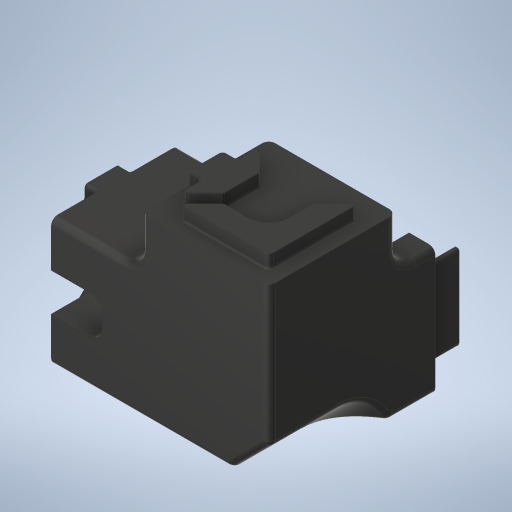
# Autodesk Inventor part: Exterior Frame Corner
Saved by Autodesk Inventor 2024 (Build 280153000, 153)
## iProperties
Category: PARTsolutions
Company: MISUMI
Created: 2024-08-20
Part Number: Exterior Frame Corner
Material: ABS Plastic
Catalog Web Link: www.cadenas.de
Description: NFS5-2020, NFSB5-2020, HFS5-2020, HFSB5-2020, CAF5-2020, HFSY5-2020, NFSF5-2020, HFSF5-2020, HFSFB5-2020, NFST5-2020, HFST5-2020, HFSTB5-2020, HFSH5-2020, HFSC5-2020-HFS5 Series Aluminum Extrusions 20 Square -1 Slot-
Vendor: MISUMI
Document SubType Name: Modeling
Designer: psAdmin
Manufacturer: MISUMI
Mass: 240.688 g
Surface Area: 837.523 cm^2
Volume: 89.1436 cm^3
Density: 1.06 g/cm^3
Appearance: Smooth - Black
PSOL_IDENT_0: {$CADENAS_DATA/23d-libs/misumi/metric/38_al_extrusions_blackets/5/hfs5_2020.prj},681 {VTYP=3D},{NB=H
PSOL_IDENT_1: FSTB5-2020-456},{LINA=HFSTB5-2020-456},{NN=NFS5-2020, NFSB5-2020, HFS5-2020, HFSB5-2020, CAF5-2020,
PSOL_IDENT_2: HFSY5-2020, NFSF5-2020, HFSF5-2020, HFSFB5-2020, NFST5-2020, HFST5-2020, HFSTB5-2020, HFSH5-2020, HF
PSOL_IDENT_3: SC5-2020},{DATE=08.05.2023 08:39:06},{GEOMDATE=27.07.2021 03:20:00},{VERSION=},{LINEID=110},{WBVAR=L
PSOL_IDENT_4: ,ALT1,ALT2,ALT4,ALT5,CP5,DL5,DR5,ALT6,ALT9,ALT10,ALT11,HP6,NHL6,DL6,NHR6,DR6,ALT7,ALT8,NH9,AH,BH,CH,
PSOL_IDENT_5: DH,EH,NH10,AV,BV,CV,DV,EV,NH11,AP,BP,CP,DP,EP,ALT12,ALT13,Z,NH12,XA,XB,XC,XD,XE,NH13,YA,YB,YC,YD,YE,
PSOL_IDENT_6: ALT16,HP16,DL16,DR16,ALT17,HQ17,JLP,ALT20},{WBNUMERIC=L,NH9,AH,BH,CH,DH,EH,NH10,AV,BV,CV,DV,EV,NH11,
PSOL_IDENT_7: AP,BP,CP,DP,EP,NH12,XA,XB,XC,XD,XE,NH13,YA,YB,YC,YD,YE,HQ17,JLP}  {NB=HFSTB5-2020-456},{LINA=HFSTB5-
PSOL_IDENT_8: 2020-456},{KT=DUMMY},{PN=HFSTB5-2020-456},{TPS=HFSTB5-2020},{MAT=A6N01SS-T5 Aluminum Alloy or 6005A-
PSOL_IDENT_9: T5 Aluminum Alloy},{ST=Black Anodize},{FRMW=20},{FRMH=20},{FRD=4.2},{L=456},{MASS=0.53},{SA=196},{LX=
PSOL_IDENT_10: 0.808x10^4},{LY=0.808x10^4},{ALT1=},{M1=0},{DPL1=0},{DPR1=0},{ALT1PN=},{ALT2=},{ALT2ALG= '','w/o End
PSOL_IDENT_11: Tapping (Heli-Coil Insert)','LHP','with LHP (Tapping on the Left (Heli-Coil Insert))','RHP','with R
PSOL_IDENT_12: HP (Tapping on the Right (Heli-Coil Insert))','HPW','with HPW (Tapping on Both Ends (Heli-Coil Inser
PSOL_IDENT_13: t))' },{M2=0},{DP2=0},{ALT2PN=},{ALT4=},{ALT4ALG= '', 'w/o SC (High Precision Cut)', 'SC', 'with SC
PSOL_IDENT_14: (High Precision Cut)' },{ALT4PN=},{ALT5=},{ALT5ALG= '','w/o 45 Degree Cut','1','with 45 Degree Cut'
PSOL_IDENT_15: },{CP5=},{CP5ALG= '','N/A' },{DL5=},{DL5ALG= '','N/A' },{DR5=},{DR5ALG= '','N/A' },{FRMLALT5=0},{FRM
PSOL_IDENT_16: RALT5=0},{ALT5PN=},{ALT6=},{ALT6ALG= '','w/o Fastening Location Wrench Access Hole Alterations','1','
PSOL_IDENT_17: with Fastening Location Wrench Access Hole Alterations' },{ALT9=},{ALT9ALG= '','w/o Location Specifi
PSOL_IDENT_18: ed Wrench Access Hole Alteratons (Horizontal)','1','with Location Specified Wrench Access Hole Alter
PSOL_IDENT_19: atons (Horizontal)' },{ALT10=},{ALT10ALG= '','w/o Location Specified Wrench Access Hole Alteratons (
PSOL_IDENT_20: Vertical)','1','with Location Specified Wrench Access Hole Alteratons (Vertical)' },{ALT11=},{ALT11A
PSOL_IDENT_21: LG= '','w/o Location Specified Wrench Access Hole Alteratons (Crisscross)','1','with Location Specif
PSOL_IDENT_22: ied Wrench Access Hole Alteratons (Crisscross)' },{HP6=},{HP6ALG= '','N/A' },{NHL6=},{NHL6ALG= '','N
PSOL_IDENT_23: /A' },{DL6=},{DL6ALG= '','N/A' },{NHR6=},{NHR6ALG= '','N/A' },{DR6=},{DR6ALG= '','N/A' },{HL6=0.000}
PSOL_IDENT_24: ,{HL6D=0},{HR6=0.000},{HR6D=0},{J6=0},{J6D=0},{K6=0},{K6D=0},{DD6=0.00},{DD6ALG=0},{ALT7=},{ALT7ALG=
PSOL_IDENT_25: '','N/A' },{ALT8=},{ALT8ALG= '','N/A' },{ALT678PN=},{NH9=0},{NH9MAX=5},{NH9ALG=[0]},{AH=0.0},{AHMIN=
PSOL_IDENT_26: 7},{AHMAX=451},{AHALG=[0]},{BH=0.0},{BHMIN=2},{BHMAX=453},{BHALG=[0]},{CH=0.0},{CHMIN=2},{CHMAX=455}
PSOL_IDENT_27: ,{CHALG=[0]},{DH=0.0},{DHMIN=2},{DHMAX=457},{DHALG=[0]},{EH=0.0},{EHMIN=2},{EHMAX=449},{EHALG=[0]},{
PSOL_IDENT_28: NH10=0},{NH10MAX=5},{NH10ALG=[0]},{AV=0.0},{AVMIN=7},{AVMAX=451},{AVALG=[0]},{BV=0.0},{BVMIN=2},{BVM
PSOL_IDENT_29: AX=453},{BVALG=[0]},{CV=0.0},{CVMIN=2},{CVMAX=455},{CVALG=[0]},{DV=0.0},{DVMIN=2},{DVMAX=457},{DVALG=
PSOL_IDENT_30: [0]},{EV=0.0},{EVMIN=2},{EVMAX=449},{EVALG=[0]},{NH11=0},{NH11MAX=5},{NH11ALG=[0]},{AP=0.0},{APMIN=7
PSOL_IDENT_31: },{APMAX=451},{APALG=[0]},{BP=0.0},{BPMIN=2},{BPMAX=453},{BPALG=[0]},{CP=0.0},{CPMIN=2},{CPMAX=455},
PSOL_IDENT_32: {CPALG=[0]},{DP=0.0},{DPMIN=2},{DPMAX=457},{DPALG=[0]},{EP=0.0},{EPMIN=2},{EPMAX=449},{EPALG=[0]},{A
PSOL_IDENT_33: LT9PN=},{ALT10PN=},{ALT11PN=},{ALT91011PN=},{ALT12=},{ALT12ALG= '','w/o Counterbore Hole in Specifie
PSOL_IDENT_34: d Position (Vertical)','1','with Counterbore Hole in Specified Position (Vertical)' },{ALT13=},{ALT1
PSOL_IDENT_35: 3ALG= '','N/A' },{Z=},{ZALG= '','N/A' },{DD12=0.0},{DD112=0.0},{NH12=0},{NH12MAX=5},{NH12ALG=[0]},{X
PSOL_IDENT_36: A=0.0},{XAMIN=7},{XAMAX=451},{XAALG=[0]},{XB=0.0},{XBMIN=2},{XBMAX=453},{XBALG=[0]},{XC=0.0},{XCMIN=
PSOL_IDENT_37: 2},{XCMAX=455},{XCALG=[0]},{XD=0.0},{XDMIN=2},{XDMAX=457},{XDALG=[0]},{XE=0.0},{XEMIN=2},{XEMAX=449}
PSOL_IDENT_38: ,{XEALG=[0]},{NH13=0},{NH13MAX=5},{NH13ALG=[0]},{YA=0.0},{YAMIN=7},{YAMAX=451},{YAALG=[0]},{YB=0.0},
PSOL_IDENT_39: {YBMIN=2},{YBMAX=453},{YBALG=[0]},{YC=0.0},{YCMIN=2},{YCMAX=455},{YCALG=[0]},{YD=0.0},{YDMIN=2},{YDM
PSOL_IDENT_40: AX=457},{YDALG=[0]},{YE=0.0},{YEMIN=2},{YEMAX=449},{YEALG=[0]},{ALT12PN=},{ALT13PN=},{ALT1213PN=},{A
PSOL_IDENT_41: LT16=},{ALT16ALG= '','w/o M Type Hole Alteration','1','with M Type Hole Alteration' },{HP16=},{HP16A
PSOL_IDENT_42: LG= '','N/A' },{DL16=},{DL16ALG= '','N/A' },{DR16=},{DR16ALG= '','N/A' },{H116=0},{D16=0.0},{ALT16PN=
PSOL_IDENT_43: },{ALT17=},{ALT17ALG= '','w/o L Type Hole Alteration (Top)','1','with L Type Hole Alteration (Top)'
PSOL_IDENT_44: },{HQ17=0},{HQ17ALG=0},{JLP=0},{JLPMIN=4.9},{JLPMAX=0},{JLPALG=[0]},{L17=0},{D17=0.0},{ALT17PN=},{AL
PSOL_IDENT_45: T20=},{ALT20PN=},{ERRORALT01=OK},{ERRORALT02=OK},{ERRORALT05=OK},{ERRORALT06091=OK},{ERRORALT06092=O
PSOL_IDENT_46: K},{ERRORALT06093=OK},{ERRORALT06094=OK},{ERRORALT06101=OK},{ERRORALT06102=OK},{ERRORALT06103=OK},{E
PSOL_IDENT_47: RRORALT06104=OK},{ERRORALT06111=OK},{ERRORALT06112=OK},{ERRORALT06113=OK},{ERRORALT06114=OK},{ERRORA
PSOL_IDENT_48: LT06121=OK},{ERRORALT06122=OK},{ERRORALT06123=OK},{ERRORALT06124=OK},{ERRORALT06131=OK},{ERRORALT061
PSOL_IDENT_49: 32=OK},{ERRORALT06133=OK},{ERRORALT06134=OK},{ERRORALT0616=OK},{ERRORALT06171=OK},{ERRORALT06172=OK}
PSOL_IDENT_50: ,{ERRORALT06173=OK},{ERRORALT0911=OK},{ERRORALT0913=OK},{ERRORALT0916=OK},{ERRORALT0917=OK},{ERRORAL
PSOL_IDENT_51: T1011=OK},{ERRORALT1012=OK},{ERRORALT1016=OK},{ERRORALT1017=OK},{ERRORALT1112=OK},{ERRORALT1113=OK},
PSOL_IDENT_52: {ERRORALT1116=OK},{ERRORALT1117=OK},{ERRORALT1216=OK},{ERRORALT1217=OK},{ERRORALT1316=OK},{ERRORALT1
PSOL_IDENT_53: 317=OK},{ERRORALT1617=OK},{ERRORPN=},{TFW=5}
NB: HFSTB5-2020-456
NN: NFS5-2020, NFSB5-2020, HFS5-2020, HFSB5-2020, CAF5-2020, HFSY5-2020, NFSF5-2020, HFSF5-2020, HFSFB5-2020, NFST5-2020, HFST5-2020, HFSTB5-2020, HFSH5-2020, HFSC5-2020
NT: HFS5 Series Aluminum Extrusions 20 Square -1 Slot-
NBSYN: $PN.
LINA: HFSTB5-2020-456
CATALOG: Misumi
PN: HFSTB5-2020-456
TPS: HFSTB5-2020
MAT: A6N01SS-T5 Aluminum Alloy or 6005A-T5 Aluminum Alloy
ST: Black Anodize
L: 456
MASS: 0.53
SA: 196
LX: 0.808x10^4
LY: 0.808x10^4
ALT1: w/o End Tapping
M1: 0
DPL1: 0
DPR1: 0
ALT2: w/o End Tapping (Heli-Coil Insert)
M2: 0
DP2: 0
ALT4: w/o SC (High Precision Cut)
ALT5: w/o 45 Degree Cut
CP5: N/A
DL5: N/A
DR5: N/A
ALT6: w/o Fastening Location Wrench Access Hole Alterations
ALT9: w/o Location Specified Wrench Access Hole Alteratons (Horizontal)
ALT10: w/o Location Specified Wrench Access Hole Alteratons (Vertical)
ALT11: w/o Location Specified Wrench Access Hole Alteratons (Crisscross)
HP6: N/A
NHL6: N/A
DL6: N/A
NHR6: N/A
DR6: N/A
HL6D: 0
HR6D: 0
J6D: 0
K6D: 0
DD6: 0
ALT7: N/A
ALT8: N/A
NH9: 0
AH: 0
BH: 0
CH: 0
DH: 0
EH: 0
NH10: 0
AV: 0
BV: 0
CV: 0
DV: 0
EV: 0
NH11: 0
AP: 0
BP: 0
CP: 0
DP: 0
EP: 0
ALT12: w/o Counterbore Hole in Specified Position (Vertical)
ALT13: N/A
Z: N/A
DD12: 0
DD112: 0
NH12: 0
XA: 0
XB: 0
XC: 0
XD: 0
XE: 0
NH13: 0
YA: 0
YB: 0
YC: 0
YD: 0
YE: 0
ALT16: w/o M Type Hole Alteration
HP16: N/A
DL16: N/A
DR16: N/A
H116: 0
D16: 0
ALT17: w/o L Type Hole Alteration (Top)
HQ17: 0
JLP: 0
D17: 0
ALT20: w/o CW (End Face C Chamfering)
SUPPLIER: MISUMI
ARTICLENO: HFSTB5-2020-456
BOMINFO: HFSTB5-2020-456
CREATOR: CADENAS GmbH
Title: HFSTB5-2020-456
Author: Cadenas PARTsolutions
Comments: HFS5 Series Aluminum Extrusions 20 Square -1 Slot-
Autodesk Inventor part; units mm, degrees
ref_plane "YZ Plane" through (0, 0, 0) normal (1, 0, 0) x (0, 1, 0)
ref_plane "XZ Plane" through (0, 0, 0) normal (0, 1, 0) x (-1, 0, 0)
ref_plane "XY Plane" through (0, 0, 0) normal (0, 0, 1) x (1, 0, 0)
sketch "Sketch_64" plane through (0, 0, 0) normal (0, 0, 1) x (1, 0, 0)
  line L0 (-10, -3) -> (-10, -9)
  arc A0 (-10, -9) -> (-9, -10) centre (-9, -9) ccw
  line L1 (-9, -10) -> (9, -10)
  arc A1 (9, -10) -> (10, -9) centre (9, -9) ccw
  line L2 (10, -9) -> (10, 9)
  arc A2 (10, 9) -> (9, 10) centre (9, 9) ccw
  line L3 (9, 10) -> (3, 10)
  line L4 (3, 10) -> (3, 8)
  line L5 (3, 8) -> (6, 8)
  line L6 (6, 8) -> (6, 7.0607)
  line L7 (6, 7.0607) -> (2.9393, 4)
  line L8 (2.9393, 4) -> (0.5196, 4)
  line L9 (0.5196, 4) -> (0, 3.7)
  line L10 (0, 3.7) -> (-0.5196, 4)
  line L11 (-0.5196, 4) -> (-2.9393, 4)
  line L12 (-2.9393, 4) -> (-6, 7.0607)
  line L13 (-6, 7.0607) -> (-6, 8)
  line L14 (-6, 8) -> (-3, 8)
  line L15 (-3, 8) -> (-3, 10)
  line L16 (-3, 10) -> (-9, 10)
  arc A3 (-9, 10) -> (-10, 9) centre (-9, 9) ccw
  line L17 (-10, 9) -> (-10, 3)
  line L18 (-10, 3) -> (-8, 3)
  line L19 (-8, 3) -> (-8, 6)
  line L20 (-8, 6) -> (-7.0607, 6)
  line L21 (-7.0607, 6) -> (-4, 2.9393)
  line L22 (-4, 2.9393) -> (-4, 0.5196)
  line L23 (-4, 0.5196) -> (-3.7, 0)
  line L24 (-3.7, 0) -> (-4, -0.5196)
  line L25 (-4, -0.5196) -> (-4, -2.9393)
  line L26 (-4, -2.9393) -> (-7.0607, -6)
  line L27 (-7.0607, -6) -> (-8, -6)
  line L28 (-8, -6) -> (-8, -3)
  line L29 (-8, -3) -> (-10, -3)
  line L30 (-6, -7.2678) -> (-6, -7.5)
  arc A4 (-6, -7.5) -> (-5.5, -8) centre (-5.5, -7.5) ccw
  line L31 (-5.5, -8) -> (7, -8)
  arc A5 (7, -8) -> (8, -7) centre (7, -7) ccw
  line L32 (8, -7) -> (8, 5.5)
  arc A6 (8, 5.5) -> (7.5, 6) centre (7.5, 5.5) ccw
  line L33 (7.5, 6) -> (7.2678, 6)
  arc A7 (7.2678, 6) -> (6.9142, 5.8536) centre (7.2678, 5.5) ccw
  line L34 (6.9142, 5.8536) -> (4.1464, 3.0858)
  arc A8 (4.1464, 3.0858) -> (4, 2.7322) centre (4.5, 2.7322) ccw
  line L35 (4, 2.7322) -> (4, -1)
  arc A9 (1, -4) -> (4, -1) centre (1, -1) ccw
  line L36 (1, -4) -> (-2.7322, -4)
  arc A10 (-2.7322, -4) -> (-3.0858, -4.1464) centre (-2.7322, -4.5) ccw
  line L37 (-3.0858, -4.1464) -> (-5.8536, -6.9142)
  arc A11 (-5.8536, -6.9142) -> (-6, -7.2678) centre (-5.5, -7.2678) ccw
  circle A12 centre (0, 0) radius 5.65
  line L38 (5.65, -5.65) -> (-10, -5.65)
  line L39 (-10, -5.65) -> (-10, 10)
  line L40 (-10, 10) -> (5.65, 10)
  line L41 (5.65, 10) -> (5.65, -5.65)
  point P0 (4.4901, 3.4295)
  point P1 (-3.4295, -4.4901)
  point P2 (5.65, 4.5893)
  point P3 (5.65, 0)
  point P4 (0, -5.65)
  point P5 (-4.5893, -5.65)
  dimension "d14" = 11.3
  constraints: 84 end point, 24 point on circle, 15 horizontal, 14 vertical, 13 centre point, 2 collinear, 2 parallel, 2 tangent, 1 coincident, 1 perpendicular, 84 other
  measures "d14" diameter of A12
extrude "Extrusion2" add sketch "Sketch_64" along normal blind 6 contours L38 L41 L34 A7 L33 A6 L32 A5 L31 A4 L30 A11 L37 | A12 L41 L38
sketch "Sketch3" plane through (0, 0, 6) normal (0, 0, 1) x (1, 0, 0)
  line L0 (6.9142, 5.8536) -> (5.65, 4.5893) projected
  arc A0 (0, -5.65) -> (5.65, 0) centre (0, 0) ccw projected
  line L1 (-4.5893, -5.65) -> (-5.8536, -6.9142) projected
  arc A1 (-5.8536, -6.9142) -> (-6, -7.2678) centre (-5.5, -7.2678) ccw projected
  line L2 (-6, -7.2678) -> (-6, -7.5) projected
  arc A2 (-6, -7.5) -> (-5.5, -8) centre (-5.5, -7.5) ccw projected
  line L3 (-5.5, -8) -> (7, -8) projected
  arc A3 (7, -8) -> (8, -7) centre (7, -7) ccw projected
  line L4 (8, -7) -> (8, 5.5) projected
  arc A4 (8, 5.5) -> (7.5, 6) centre (7.5, 5.5) ccw projected
  line L5 (7.5, 6) -> (7.2678, 6) projected
  arc A5 (7.2678, 6) -> (6.9142, 5.8536) centre (7.2678, 5.5) ccw projected
  line L6 (5.65, 4.5893) -> (5.65, 0) projected
  line L7 (0, -5.65) -> (-4.5893, -5.65) projected
  line L8 (7, -7.75) -> (-5.5, -7.75)
  arc A6 (-5.75, -7.5) -> (-5.5, -7.75) centre (-5.5, -7.5) ccw
  line L9 (-5.75, -7.5) -> (-5.75, -7.2678)
  arc A7 (-5.6768, -7.091) -> (-5.75, -7.2678) centre (-5.5, -7.2678) ccw
  line L10 (-5.6768, -7.091) -> (-4.4858, -5.9)
  line L11 (-4.4858, -5.9) -> (0, -5.9)
  arc A8 (0, -5.9) -> (5.9, 0) centre (0, 0) ccw
  line L12 (5.9, 0) -> (5.9, 4.4858)
  line L13 (5.9, 4.4858) -> (7.091, 5.6768)
  arc A9 (7.2678, 5.75) -> (7.091, 5.6768) centre (7.2678, 5.5) ccw
  line L14 (7.2678, 5.75) -> (7.5, 5.75)
  arc A10 (7.75, 5.5) -> (7.5, 5.75) centre (7.5, 5.5) ccw
  line L15 (7.75, 5.5) -> (7.75, -7)
  arc A11 (7, -7.75) -> (7.75, -7) centre (7, -7) ccw
  dimension "d25" = 0.25
  constraints: 16 end point, 12 point on circle, 6 centre point, 13 other
  measures "d25" distance between parallel lines of L3 L8
extrude "Extrusion3" cut sketch "Sketch3" against normal through all
sketch "Sketch4" plane through (0, 0, 6) normal (0, 0, 1) x (1, 0, 0)
  line L0 (-9, 10) -> (9, 10)
  line L1 (10, 9) -> (10, -9)
  line L2 (9, -10) -> (-9, -10)
  line L3 (-10, -9) -> (-10, 9)
  line L4 (-10, 10) -> (10, -10) construction
  line L5 (10, 10) -> (-10, -10) construction
  arc A0 (9, -10) -> (10, -9) centre (9, -9) ccw
  arc A1 (-10, -9) -> (-9, -10) centre (-9, -9) ccw
  arc A2 (-9, 10) -> (-10, 9) centre (-9, 9) ccw
  arc A3 (10, 9) -> (9, 10) centre (9, 9) ccw
  arc A4 (7, -7.75) -> (7.75, -7) centre (7, -7) ccw projected
  line L6 (7.75, -7) -> (7.75, 5.5) projected
  arc A5 (7.75, 5.5) -> (7.5, 5.75) centre (7.5, 5.5) ccw projected
  line L7 (7.5, 5.75) -> (7.2678, 5.75) projected
  arc A6 (7.2678, 5.75) -> (7.091, 5.6768) centre (7.2678, 5.5) ccw projected
  line L8 (7.091, 5.6768) -> (5.9, 4.4858) projected
  line L9 (5.9, 4.4858) -> (5.9, 0) projected
  arc A7 (0, -5.9) -> (5.9, 0) centre (0, 0) ccw projected
  line L10 (0, -5.9) -> (-4.4858, -5.9) projected
  line L11 (-4.4858, -5.9) -> (-5.6768, -7.091) projected
  arc A8 (-5.6768, -7.091) -> (-5.75, -7.2678) centre (-5.5, -7.2678) ccw projected
  line L12 (-5.75, -7.2678) -> (-5.75, -7.5) projected
  arc A9 (-5.75, -7.5) -> (-5.5, -7.75) centre (-5.5, -7.5) ccw projected
  line L13 (-5.5, -7.75) -> (7, -7.75) projected
  line L14 (5.9, 4.4858) -> (5.9, 10)
  line L15 (-4.4858, -5.9) -> (-10, -5.9)
  dimension "d21" = 1
  dimension "d22" = 20
  dimension "d23" = 20
  dimension "d24" = 1
  constraints: 16 end point, 10 point on line, 8 point on circle, 8 tangent, 4 centre point, 3 perpendicular, 2 equal radius, 2 midpoint, 2 parallel, 1 horizontal
  measures "d21" radius of A0
  measures "d22" distance between parallel lines of L3 L1
  measures "d23" distance between parallel lines of L0 L2
  measures "d24" radius of A1
extrude "Extrusion4" add sketch "Sketch4" along normal blind 6.15 contours L0 A3 L1 A0 L2 A1 L3 L15 L11 A8 L12 A9 L13 A4 L6 A5 L7 A6 L8 L14 | L8 A6 L7 A5 L6 A4 L13 A9 L12 A8 L11 L10 A7 L9
ref_plane "Work Plane4" through (0, 0, 32.15) normal (0, 0, -1) x (-1, 0, 0)
extrude "Extrusion5" add sketch "Sketch4" along normal up to surface (20 mm away) from surface at 6.15
ref_plane "Work Plane5" through (5.9, 17.8, 6) normal (0, 1, 0) x (1, 0, 0)
sketch "Sketch5" plane through (5.9, 17.8, 6) normal (0, 1, 0) x (1, 0, 0)
  line L0 (4.1, 0) -> (4.1, -26.15) projected
  line L1 (3.1, -26.15) -> (-14.9, -26.15) projected
  line L2 (-15.9, -6.15) -> (4.1, -6.15)
  line L3 (4.1, -6.15) -> (4.1, -26.15)
  line L4 (4.1, -26.15) -> (-15.9, -26.15)
  line L5 (-15.9, -26.15) -> (-15.9, -6.15)
  line L6 (-15.9, -6.15) -> (4.1, -26.15) construction
  line L7 (4.1, -6.15) -> (-15.9, -26.15) construction
  point P0 (-5.9, 6)
  point P1 (-5.9, -16.15)
  point P2 (4.1, -6.15)
  dimension "d32" = 20
  dimension "d33" = 20
  constraints: 12 end point, 2 collinear, 2 midpoint, 2 parallel, 1 horizontal, 1 perpendicular
  measures "d32" distance of L3.end L4.end
  measures "d33" distance of L2.end L3.end
extrude "Extrusion6" add sketch "Sketch5" against normal blind 18
ref_plane "Work Plane6" through (-24.15, -9, 6) normal (-1, 0, 0) x (0, 0, 1)
sketch "Sketch6" plane through (-24.15, -9, 6) normal (-1, 0, 0) x (0, 0, 1)
  line L0 (6.15, 3.1) -> (6.15, 26.8) projected
  line L1 (0, 3.1) -> (6.15, 3.1) projected
  line L2 (0, 3.1) -> (0, 0) projected
  line L3 (0, 0) -> (26.15, 0) projected
  line L4 (26.15, 26.8) -> (26.15, 0) projected
  line L5 (6.15, 26.8) -> (26.15, 26.8) projected
  line L6 (0, -1) -> (26.15, -1) projected
  line L7 (26.15, -1) -> (26.15, 0) projected
  line L8 (6.15, 19) -> (26.15, 19)
  line L9 (26.15, 19) -> (26.15, -1)
  line L10 (26.15, -1) -> (6.15, -1)
  line L11 (6.15, -1) -> (6.15, 19)
  line L12 (6.15, 19) -> (26.15, -1) construction
  line L13 (26.15, 19) -> (6.15, -1) construction
  point P0 (-6, 9)
  point P1 (16.15, 9)
  point P2 (6.15, -1)
  point P3 (26.15, 19)
  point P4 (6.15, 19)
  dimension "d37" = 20
  dimension "d38" = 20
  constraints: 12 end point, 2 midpoint, 2 parallel, 1 horizontal, 1 perpendicular
  measures "d37" distance of L6.end L10.end
  measures "d38" distance of L6.end L8.end
extrude "Extrusion7" add sketch "Sketch6" against normal blind 24.35 contours L0 L8 L4 L3 L11 | L3 L7 L6 L11
sketch "Sketch7" plane through (-10, 17.8, 32.15) normal (0, 0, 1) x (1, 0, 0)
  line L0 (-14.15, -7.8) -> (0, -7.8) projected
  line L1 (-14.15, -27.8) -> (-14.15, -7.8) projected
  line L2 (-14.15, -27.8) -> (19, -27.8) projected
  arc A0 (19, -27.8) -> (20, -26.8) centre (19, -26.8) ccw projected
  line L3 (20, 0) -> (20, -26.8) projected
  line L4 (0, 0) -> (20, 0) projected
  line L5 (0, 0) -> (0, -7.8) projected
  line L6 (20, -21.8) -> (14, -27.8)
  point P0 (10, -17.8)
  dimension "d41" = 6
  dimension "d42" = 6
  constraints: 2 end point, 2 point on line
  measures "d41" distance from line of L2 L6.start
  measures "d42" distance from line of L6.end L3
extrude "Extrusion8" cut sketch "Sketch7" against normal blind 15 contours L6 L3 A0 L2
ref_plane "Work Plane7" through (10, -4, 17.15) normal (0.5, -0.5, 0.7071068) x (0.7071068, 0.7071068, 0)
sketch "Sketch8" plane through (-10, 17.8, 17.15) normal (0, 0, 1) x (1, 0, 0)
  line L0 (20, -21.8) -> (20, -26.8) projected
  line L1 (14, -27.8) -> (20, -21.8) projected
  line L2 (19, -27.8) -> (14, -27.8) projected
  arc A0 (19, -27.8) -> (20, -26.8) centre (19, -26.8) ccw projected
  point P0 (10, -17.8)
extrude "Extrusion9" cut sketch "Sketch8" along normal up to surface surface through (10, -4, 17.15) normal (0.5, -0.5, 0.7071068)
fillet "Fillet1" radius 10 1 edges at (7, -7, 17.15)
sketch "Sketch9" plane through (0, 0, 6) normal (0, 0, -1) x (-1, 0, 0)
  line L0 (-7.091, 5.6768) -> (-5.9, 4.4858) projected
  line L1 (-5.9, 10) -> (-5.9, 4.4858) projected
  line L2 (-9, 10) -> (-5.9, 10) projected
  arc A0 (-9, 10) -> (-10, 9) centre (-9, 9) ccw projected
  line L3 (-10, -9) -> (-10, 9) projected
  arc A1 (-10, -9) -> (-9, -10) centre (-9, -9) ccw projected
  line L4 (9, -10) -> (-9, -10) projected
  arc A2 (9, -10) -> (10, -9) centre (9, -9) ccw projected
  line L5 (10, -5.9) -> (10, -9) projected
  line L6 (4.4858, -5.9) -> (10, -5.9) projected
  line L7 (4.4858, -5.9) -> (5.6768, -7.091) projected
  arc A3 (5.75, -7.2678) -> (5.6768, -7.091) centre (5.5, -7.2678) ccw projected
  line L8 (5.75, -7.2678) -> (5.75, -7.5) projected
  arc A4 (5.5, -7.75) -> (5.75, -7.5) centre (5.5, -7.5) ccw projected
  line L9 (5.5, -7.75) -> (-7, -7.75) projected
  arc A5 (-7.75, -7) -> (-7, -7.75) centre (-7, -7) ccw projected
  line L10 (-7.75, -7) -> (-7.75, 5.5) projected
  arc A6 (-7.5, 5.75) -> (-7.75, 5.5) centre (-7.5, 5.5) ccw projected
  line L11 (-7.5, 5.75) -> (-7.2678, 5.75) projected
  arc A7 (-7.091, 5.6768) -> (-7.2678, 5.75) centre (-7.2678, 5.5) ccw projected
  line L12 (10, 10) -> (-10, 10)
  line L13 (-10, 10) -> (-10, -10)
  line L14 (-10, -10) -> (10, -10)
  line L15 (10, -10) -> (10, 10)
  line L16 (10, 10) -> (-10, -10) construction
  line L17 (-10, 10) -> (10, -10) construction
  point P0 (0, 0)
  point P1 (10, -9)
  point P2 (-10, 9)
  constraints: 12 end point, 2 collinear, 2 midpoint, 2 parallel, 1 horizontal, 1 perpendicular
extrude "Extrusion10" add sketch "Sketch9" against normal up to surface (6.15 mm away) contours A0 L13 L12 | L15 L14 A2
fillet "Fillet2" radius 3 1 edges at (-10, 10, 22.15)
fillet "Fillet3" radius 1 7 edges at (10, -5.0765, 17.4653) (10, -8.5711, 13.9178) (9.7071, -9.7071, 13.3216) (8.5711, -10, 13.9178) (5.0765, -10, 17.4653) (4, -10, 26.7211) (10, -4, 26.7211)
fillet "Fillet4" radius 3 2 edges at (-10, -7.95, 12.15) (7.95, 10, 12.15)
fillet "Fillet5" radius 1 17 edges at (-10.8787, -10, 11.2713) (-10, -10, 7.575) (-18.575, -10, 12.15) (10, 10.8787, 11.2713) (10, 10, 7.575) (10, 15.4, 12.15) (9.9239, -3.9685, 32.15) (7, -7, 32.15) (3.9685, -9.9239, 32.15) (-10.2821, -10, 32.15) (10, 7.1071, 32.15) (-10, 15.4, 32.15) (-18.575, 10, 32.15) (-10.8787, 10.8787, 32.15) (-10.8787, 10.8787, 12.15) (-10, 15.4, 12.15) (-18.575, 10, 12.15)
sketch "Sketch10" plane through (-24.15, -9, 6) normal (-1, 0, 0) x (0, 0, 1)
  circle A0 centre (16.15, 9) radius 2.1 projected
  arc A1 (21.65, 1) -> (22.15, 1.5) centre (21.65, 1.5) ccw projected
  line L0 (21.65, 1) -> (10.65, 1) projected
  arc A2 (10.15, 1.5) -> (10.65, 1) centre (10.65, 1.5) ccw projected
  line L1 (10.15, 1.5) -> (10.15, 1.7322) projected
  arc A3 (10.2964, 2.0858) -> (10.15, 1.7322) centre (10.65, 1.7322) ccw projected
  line L2 (10.2964, 2.0858) -> (13.0642, 4.8536) projected
  arc A4 (13.4178, 5) -> (13.0642, 4.8536) centre (13.4178, 4.5) ccw projected
  line L3 (13.4178, 5) -> (18.8822, 5) projected
  arc A5 (19.2358, 4.8536) -> (18.8822, 5) centre (18.8822, 4.5) ccw projected
  line L4 (19.2358, 4.8536) -> (22.0036, 2.0858) projected
  arc A6 (22.15, 1.7322) -> (22.0036, 2.0858) centre (21.65, 1.7322) ccw projected
  line L5 (22.15, 1.7322) -> (22.15, 1.5) projected
  line L6 (26.15, 0) -> (26.15, 6) projected
  line L7 (26.15, 6) -> (24.15, 6) projected
  line L8 (24.15, 6) -> (24.15, 3) projected
  line L9 (24.15, 3) -> (23.2107, 3) projected
  line L10 (23.2107, 3) -> (20.15, 6.0607) projected
  line L11 (20.15, 6.0607) -> (20.15, 8.4804) projected
  line L12 (20.15, 8.4804) -> (19.85, 9) projected
  line L13 (19.85, 9) -> (20.15, 9.5196) projected
  line L14 (20.15, 9.5196) -> (20.15, 11.9393) projected
  line L15 (20.15, 11.9393) -> (23.2107, 15) projected
  line L16 (23.2107, 15) -> (24.15, 15) projected
  line L17 (24.15, 15) -> (24.15, 12) projected
  line L18 (24.15, 12) -> (26.15, 12) projected
  line L19 (26.15, 12) -> (26.15, 18) projected
  arc A7 (26.15, 18) -> (25.15, 19) centre (25.15, 18) ccw projected
  line L20 (25.15, 19) -> (19.15, 19) projected
  line L21 (19.15, 19) -> (19.15, 17) projected
  line L22 (19.15, 17) -> (22.15, 17) projected
  line L23 (22.15, 17) -> (22.15, 16.0607) projected
  line L24 (22.15, 16.0607) -> (19.0893, 13) projected
  line L25 (19.0893, 13) -> (16.6696, 13) projected
  line L26 (16.6696, 13) -> (16.15, 12.7) projected
  line L27 (16.15, 12.7) -> (15.6304, 13) projected
  line L28 (15.6304, 13) -> (13.2107, 13) projected
  line L29 (13.2107, 13) -> (10.15, 16.0607) projected
  line L30 (10.15, 16.0607) -> (10.15, 17) projected
  line L31 (10.15, 17) -> (13.15, 17) projected
  line L32 (13.15, 17) -> (13.15, 19) projected
  line L33 (13.15, 19) -> (7.15, 19) projected
  arc A8 (7.15, 19) -> (6.15, 18) centre (7.15, 18) ccw projected
  line L34 (6.15, 18) -> (6.15, 12) projected
  line L35 (6.15, 12) -> (8.15, 12) projected
  line L36 (8.15, 12) -> (8.15, 15) projected
  line L37 (8.15, 15) -> (9.0893, 15) projected
  line L38 (9.0893, 15) -> (12.15, 11.9393) projected
  line L39 (12.15, 11.9393) -> (12.15, 9.5196) projected
  line L40 (12.15, 9.5196) -> (12.45, 9) projected
  line L41 (12.45, 9) -> (12.15, 8.4804) projected
  line L42 (12.15, 8.4804) -> (12.15, 6.0607) projected
  line L43 (12.15, 6.0607) -> (9.0893, 3) projected
  line L44 (9.0893, 3) -> (8.15, 3) projected
  line L45 (8.15, 3) -> (8.15, 6) projected
  line L46 (8.15, 6) -> (6.15, 6) projected
  line L47 (6.15, 6) -> (6.15, 0) projected
  arc A9 (6.15, 0) -> (7.15, -1) centre (7.15, 0) ccw projected
  line L48 (7.15, -1) -> (25.15, -1) projected
  arc A10 (25.15, -1) -> (26.15, 0) centre (25.15, 0) ccw projected
  line L49 (26.15, 6) -> (20.15, 6)
  line L50 (20.15, 6) -> (20.15, 11.9393)
  line L51 (20.15, 11.9393) -> (26.15, 11.9393)
  line L52 (26.15, 11.9393) -> (26.15, 6)
  line L53 (13.15, 19) -> (19.15, 19)
  line L54 (16.6696, 13) -> (15.6304, 13)
  point P0 (-6, 9)
  point P1 (20.2107, 6)
  constraints: 12 end point, 3 equal length, 2 horizontal, 1 perpendicular
sketch "Sketch11" plane through (5.9, 17.8, 6) normal (0, 1, 0) x (1, 0, 0)
  circle A0 centre (-5.9, -16.15) radius 2.1 projected
  arc A1 (-11.7536, -23.0642) -> (-11.9, -23.4178) centre (-11.4, -23.4178) ccw projected
  line L0 (-11.9, -23.4178) -> (-11.9, -23.65) projected
  arc A2 (-11.9, -23.65) -> (-11.4, -24.15) centre (-11.4, -23.65) ccw projected
  line L1 (-11.4, -24.15) -> (1.1, -24.15) projected
  arc A3 (1.1, -24.15) -> (2.1, -23.15) centre (1.1, -23.15) ccw projected
  line L2 (2.1, -23.15) -> (2.1, -10.65) projected
  arc A4 (2.1, -10.65) -> (1.6, -10.15) centre (1.6, -10.65) ccw projected
  line L3 (1.6, -10.15) -> (1.3678, -10.15) projected
  arc A5 (1.3678, -10.15) -> (1.0142, -10.2964) centre (1.3678, -10.65) ccw projected
  line L4 (1.0142, -10.2964) -> (-1.7536, -13.0642) projected
  arc A6 (-1.7536, -13.0642) -> (-1.9, -13.4178) centre (-1.4, -13.4178) ccw projected
  line L5 (-1.9, -13.4178) -> (-1.9, -17.15) projected
  arc A7 (-4.9, -20.15) -> (-1.9, -17.15) centre (-4.9, -17.15) ccw projected
  line L6 (-4.9, -20.15) -> (-8.6322, -20.15) projected
  arc A8 (-8.6322, -20.15) -> (-8.9858, -20.2964) centre (-8.6322, -20.65) ccw projected
  line L7 (-8.9858, -20.2964) -> (-11.7536, -23.0642) projected
  line L8 (-15.9, -25.15) -> (-15.9, -19.15) projected
  line L9 (-15.9, -19.15) -> (-13.9, -19.15) projected
  line L10 (-13.9, -19.15) -> (-13.9, -22.15) projected
  line L11 (-13.9, -22.15) -> (-12.9607, -22.15) projected
  line L12 (-12.9607, -22.15) -> (-9.9, -19.0893) projected
  line L13 (-9.9, -19.0893) -> (-9.9, -16.6696) projected
  line L14 (-9.9, -16.6696) -> (-9.6, -16.15) projected
  line L15 (-9.6, -16.15) -> (-9.9, -15.6304) projected
  line L16 (-9.9, -15.6304) -> (-9.9, -13.2107) projected
  line L17 (-9.9, -13.2107) -> (-12.9607, -10.15) projected
  line L18 (-12.9607, -10.15) -> (-13.9, -10.15) projected
  line L19 (-13.9, -10.15) -> (-13.9, -13.15) projected
  line L20 (-13.9, -13.15) -> (-15.9, -13.15) projected
  line L21 (-15.9, -13.15) -> (-15.9, -7.15) projected
  arc A9 (-14.9, -6.15) -> (-15.9, -7.15) centre (-14.9, -7.15) ccw projected
  line L22 (-14.9, -6.15) -> (-8.9, -6.15) projected
  line L23 (-8.9, -6.15) -> (-8.9, -8.15) projected
  line L24 (-8.9, -8.15) -> (-11.9, -8.15) projected
  line L25 (-11.9, -8.15) -> (-11.9, -9.0893) projected
  line L26 (-11.9, -9.0893) -> (-8.8393, -12.15) projected
  line L27 (-8.8393, -12.15) -> (-6.4196, -12.15) projected
  line L28 (-6.4196, -12.15) -> (-5.9, -12.45) projected
  line L29 (-5.9, -12.45) -> (-5.3804, -12.15) projected
  line L30 (-5.3804, -12.15) -> (-2.9607, -12.15) projected
  line L31 (-2.9607, -12.15) -> (0.1, -9.0893) projected
  line L32 (0.1, -9.0893) -> (0.1, -8.15) projected
  line L33 (0.1, -8.15) -> (-2.9, -8.15) projected
  line L34 (-2.9, -8.15) -> (-2.9, -6.15) projected
  line L35 (-2.9, -6.15) -> (3.1, -6.15) projected
  arc A10 (4.1, -7.15) -> (3.1, -6.15) centre (3.1, -7.15) ccw projected
  line L36 (4.1, -7.15) -> (4.1, -25.15) projected
  arc A11 (3.1, -26.15) -> (4.1, -25.15) centre (3.1, -25.15) ccw projected
  line L37 (3.1, -26.15) -> (-14.9, -26.15) projected
  arc A12 (-15.9, -25.15) -> (-14.9, -26.15) centre (-14.9, -25.15) ccw projected
  line L38 (-15.9, -19.15) -> (-15.9, -13.15)
  line L39 (-15.9, -25.15) -> (-15.9, -7.15) projected
  line L40 (-2.9, -6.15) -> (-8.9, -6.15)
  line L41 (-5.9, -6.15) -> (-18.9, -6.15) projected
  line L42 (-9.9, -15.6304) -> (-9.9, -16.6696)
  point P0 (-5.9, 6)
  constraints: 6 end point, 2 collinear
sketch "Sketch12" plane through (-24.15, -9, 6) normal (-1, 0, 0) x (0, 0, 1)
  arc A0 (7.15, 19) -> (6.15, 18) centre (7.15, 18) ccw projected
  line L0 (6.15, 18) -> (6.15, 0) projected
  arc A1 (6.15, 0) -> (7.15, -1) centre (7.15, 0) ccw projected
  line L1 (7.15, -1) -> (25.15, -1) projected
  arc A2 (25.15, -1) -> (26.15, 0) centre (25.15, 0) ccw projected
  line L2 (26.15, 0) -> (26.15, 18) projected
  arc A3 (26.15, 18) -> (25.15, 19) centre (25.15, 18) ccw projected
  line L3 (25.15, 19) -> (7.15, 19) projected
  line L4 (19.2358, 4.8536) -> (22.0036, 2.0858) projected
  arc A4 (22.15, 1.7322) -> (22.0036, 2.0858) centre (21.65, 1.7322) ccw projected
  line L5 (22.15, 1.7322) -> (22.15, 1.5) projected
  arc A5 (21.65, 1) -> (22.15, 1.5) centre (21.65, 1.5) ccw projected
  line L6 (21.65, 1) -> (10.65, 1) projected
  arc A6 (10.15, 1.5) -> (10.65, 1) centre (10.65, 1.5) ccw projected
  line L7 (10.15, 1.5) -> (10.15, 1.7322) projected
  arc A7 (10.2964, 2.0858) -> (10.15, 1.7322) centre (10.65, 1.7322) ccw projected
  line L8 (10.2964, 2.0858) -> (13.0642, 4.8536) projected
  arc A8 (13.4178, 5) -> (13.0642, 4.8536) centre (13.4178, 4.5) ccw projected
  line L9 (13.4178, 5) -> (18.8822, 5) projected
  arc A9 (19.2358, 4.8536) -> (18.8822, 5) centre (18.8822, 4.5) ccw projected
  line L10 (22.15, 17) -> (22.15, 16.0607) projected
  line L11 (22.15, 16.0607) -> (19.0893, 13) projected
  line L12 (19.0893, 13) -> (16.6696, 13) projected
  line L13 (16.6696, 13) -> (16.15, 12.7) projected
  line L14 (16.15, 12.7) -> (15.6304, 13) projected
  line L15 (15.6304, 13) -> (13.2107, 13) projected
  line L16 (13.2107, 13) -> (10.15, 16.0607) projected
  line L17 (10.15, 16.0607) -> (10.15, 17) projected
  line L18 (10.15, 17) -> (13.15, 17) projected
  line L19 (13.15, 17) -> (13.15, 19) projected
  line L20 (19.15, 19) -> (19.15, 17) projected
  line L21 (19.15, 17) -> (22.15, 17) projected
  line L22 (16.6696, 13) -> (15.6304, 13)
  point P0 (-6, 9)
  constraints: 2 end point, 1 horizontal
extrude "Extrusion12" add sketch "Sketch12" along normal blind 2 contours L3 L20 L21 L10 L11 L12 L22 L15 L16 L17 L18 L19 | L4 A4 L5 A5 L6 A6 L7 A7 L8 A8 L9 A9
extrude "Extrusion11" cut sketch "Sketch10" against normal blind 8 contours L7 L49 L10 L11 L50 L14 L51 L52
fillet "Fillet6" radius 2 2 edges at (-16.15, -3, 29.1803) (-16.15, 2.9393, 29.15)
sketch "Sketch13" plane through (-26.15, -9, 6) normal (-1, 0, 0) x (0, 0, 1)
  line L0 (13.0642, 4.8536) -> (10.2964, 2.0858) projected
  arc A0 (10.2964, 2.0858) -> (10.15, 1.7322) centre (10.65, 1.7322) ccw projected
  line L1 (10.15, 1.7322) -> (10.15, 1.5) projected
  arc A1 (10.15, 1.5) -> (10.65, 1) centre (10.65, 1.5) ccw projected
  line L2 (10.65, 1) -> (21.65, 1) projected
  arc A2 (21.65, 1) -> (22.15, 1.5) centre (21.65, 1.5) ccw projected
  line L3 (22.15, 1.5) -> (22.15, 1.7322) projected
  arc A3 (22.15, 1.7322) -> (22.0036, 2.0858) centre (21.65, 1.7322) ccw projected
  line L4 (22.0036, 2.0858) -> (19.2358, 4.8536) projected
  arc A4 (19.2358, 4.8536) -> (18.8822, 5) centre (18.8822, 4.5) ccw projected
  line L5 (18.8822, 5) -> (13.4178, 5) projected
  arc A5 (13.4178, 5) -> (13.0642, 4.8536) centre (13.4178, 4.5) ccw projected
  line L6 (10.15, 17) -> (10.15, 16.0607) projected
  line L7 (10.15, 16.0607) -> (13.2107, 13) projected
  line L8 (13.2107, 13) -> (19.0893, 13) projected
  line L9 (19.0893, 13) -> (22.15, 16.0607) projected
  line L10 (22.15, 16.0607) -> (22.15, 17) projected
  line L11 (22.15, 17) -> (19.15, 17) projected
  line L12 (19.15, 17) -> (19.15, 19) projected
  line L13 (19.15, 19) -> (13.15, 19) projected
  line L14 (13.15, 19) -> (13.15, 17) projected
  line L15 (13.15, 17) -> (10.15, 17) projected
  line L16 (10.4732, 1.909) -> (13.241, 4.6768)
  arc A6 (13.4178, 4.75) -> (13.241, 4.6768) centre (13.4178, 4.5) ccw
  line L17 (13.4178, 4.75) -> (18.8822, 4.75)
  arc A7 (19.059, 4.6768) -> (18.8822, 4.75) centre (18.8822, 4.5) ccw
  line L18 (19.059, 4.6768) -> (21.8268, 1.909)
  arc A8 (21.9, 1.7322) -> (21.8268, 1.909) centre (21.65, 1.7322) ccw
  line L19 (21.9, 1.7322) -> (21.9, 1.5)
  arc A9 (21.65, 1.25) -> (21.9, 1.5) centre (21.65, 1.5) ccw
  line L20 (21.65, 1.25) -> (10.65, 1.25)
  arc A10 (10.4, 1.5) -> (10.65, 1.25) centre (10.65, 1.5) ccw
  line L21 (10.4, 1.5) -> (10.4, 1.7322)
  arc A11 (10.4732, 1.909) -> (10.4, 1.7322) centre (10.65, 1.7322) ccw
  line L22 (18.9858, 13.25) -> (13.3142, 13.25)
  line L23 (13.3142, 13.25) -> (10.4, 16.1642)
  line L24 (10.4, 16.1642) -> (10.4, 16.75)
  line L25 (10.4, 16.75) -> (13.4, 16.75)
  line L26 (13.4, 16.75) -> (13.4, 18.75)
  line L27 (13.4, 18.75) -> (18.9, 18.75)
  line L28 (18.9, 18.75) -> (18.9, 16.75)
  line L29 (18.9, 16.75) -> (21.9, 16.75)
  line L30 (21.9, 16.75) -> (21.9, 16.1642)
  line L31 (21.9, 16.1642) -> (18.9858, 13.25)
  line L32 (18.9, 18.75) -> (13.4, 18.75)
  line L33 (13.4, 18.75) -> (13.4, 19)
  line L34 (13.4, 19) -> (18.9, 19)
  line L35 (18.9, 19) -> (18.9, 18.75)
  line L36 (19.15, 19) -> (13.15, 19) projected
  point P0 (-6, 9)
  dimension "d61" = 0.25
  dimension "d97" = 0.25
  constraints: 40 end point, 12 point on circle, 6 centre point, 2 parallel, 1 horizontal, 1 perpendicular, 1 point on line, 20 other
  measures "d61" distance between parallel lines of L0 L16
  measures "d97" distance between parallel lines of L8 L22
extrude "Extrusion13" cut sketch "Sketch13" against normal up to surface (2 mm away) contours A5 L5 A4 L4 A3 L3 A2 L2 A1 L1 A0 L0 | L15 L14 L13 L33 L26 L25 L24 L23 L22 L31 L30 L29 L28 L35 L12 L11 L10 L9 L8 L7 L6
fillet "Fillet7" radius 0.5 10 edges at (-25.15, 7.1642, 27.9) (-25.15, 10, 24.9) (-25.15, 7.75, 24.9) (-25.15, 7.75, 19.4) (-25.15, 10, 19.4) (-25.15, 7.75, 16.4) (-25.15, 7.75, 27.9) (-25.15, 4.25, 24.9858) (-25.15, 7.1642, 16.4) (-25.15, 4.25, 19.3142)
extrude "Extrusion14" add sketch "Sketch11" along normal blind 2 contours L7 A8 L6 A7 L5 A6 L4 A5 L3 A4 L2 A3 L1 A2 L0 A1 | L38 L20 L19 L18 L17 L16 L42 L13 L12 L11 L10 L9
sketch "Sketch14" plane through (5.9, 19.8, 6) normal (0, 1, 0) x (1, 0, 0)
  line L0 (-13.9, -13.15) -> (-15.9, -13.15) projected
  line L1 (-15.9, -13.15) -> (-15.9, -19.15) projected
  line L2 (-15.9, -19.15) -> (-13.9, -19.15) projected
  line L3 (-13.9, -19.15) -> (-13.9, -22.15) projected
  line L4 (-13.9, -22.15) -> (-12.9607, -22.15) projected
  line L5 (-12.9607, -22.15) -> (-9.9, -19.0893) projected
  line L6 (-9.9, -19.0893) -> (-9.9, -13.2107) projected
  line L7 (-9.9, -13.2107) -> (-12.9607, -10.15) projected
  line L8 (-12.9607, -10.15) -> (-13.9, -10.15) projected
  line L9 (-13.9, -10.15) -> (-13.9, -13.15) projected
  arc A0 (-8.6322, -20.15) -> (-8.9858, -20.2964) centre (-8.6322, -20.65) ccw projected
  line L10 (-8.9858, -20.2964) -> (-11.7536, -23.0642) projected
  arc A1 (-11.7536, -23.0642) -> (-11.9, -23.4178) centre (-11.4, -23.4178) ccw projected
  line L11 (-11.9, -23.4178) -> (-11.9, -23.65) projected
  arc A2 (-11.9, -23.65) -> (-11.4, -24.15) centre (-11.4, -23.65) ccw projected
  line L12 (-11.4, -24.15) -> (1.1, -24.15) projected
  arc A3 (1.1, -24.15) -> (2.1, -23.15) centre (1.1, -23.15) ccw projected
  line L13 (2.1, -23.15) -> (2.1, -10.65) projected
  arc A4 (2.1, -10.65) -> (1.6, -10.15) centre (1.6, -10.65) ccw projected
  line L14 (1.6, -10.15) -> (1.3678, -10.15) projected
  arc A5 (1.3678, -10.15) -> (1.0142, -10.2964) centre (1.3678, -10.65) ccw projected
  line L15 (1.0142, -10.2964) -> (-1.7536, -13.0642) projected
  arc A6 (-1.7536, -13.0642) -> (-1.9, -13.4178) centre (-1.4, -13.4178) ccw projected
  line L16 (-1.9, -13.4178) -> (-1.9, -17.15) projected
  arc A7 (-4.9, -20.15) -> (-1.9, -17.15) centre (-4.9, -17.15) ccw projected
  line L17 (-4.9, -20.15) -> (-8.6322, -20.15) projected
  line L18 (-1.65, -17.15) -> (-1.65, -13.4178)
  arc A8 (-1.5768, -13.241) -> (-1.65, -13.4178) centre (-1.4, -13.4178) ccw
  line L19 (-1.5768, -13.241) -> (1.191, -10.4732)
  arc A9 (1.3678, -10.4) -> (1.191, -10.4732) centre (1.3678, -10.65) ccw
  line L20 (1.3678, -10.4) -> (1.6, -10.4)
  arc A10 (1.85, -10.65) -> (1.6, -10.4) centre (1.6, -10.65) ccw
  line L21 (1.85, -10.65) -> (1.85, -23.15)
  arc A11 (1.1, -23.9) -> (1.85, -23.15) centre (1.1, -23.15) ccw
  line L22 (1.1, -23.9) -> (-11.4, -23.9)
  arc A12 (-11.65, -23.65) -> (-11.4, -23.9) centre (-11.4, -23.65) ccw
  line L23 (-11.65, -23.65) -> (-11.65, -23.4178)
  arc A13 (-11.5768, -23.241) -> (-11.65, -23.4178) centre (-11.4, -23.4178) ccw
  line L24 (-11.5768, -23.241) -> (-8.809, -20.4732)
  arc A14 (-8.6322, -20.4) -> (-8.809, -20.4732) centre (-8.6322, -20.65) ccw
  line L25 (-8.6322, -20.4) -> (-4.9, -20.4)
  arc A15 (-4.9, -20.4) -> (-1.65, -17.15) centre (-4.9, -17.15) ccw
  line L26 (-10.15, -13.3142) -> (-10.15, -18.9858)
  line L27 (-10.15, -18.9858) -> (-13.0642, -21.9)
  line L28 (-13.0642, -21.9) -> (-13.65, -21.9)
  line L29 (-13.65, -21.9) -> (-13.65, -18.9)
  line L30 (-13.65, -18.9) -> (-15.65, -18.9)
  line L31 (-15.65, -18.9) -> (-15.65, -13.4)
  line L32 (-15.65, -13.4) -> (-13.65, -13.4)
  line L33 (-13.65, -13.4) -> (-13.65, -10.4)
  line L34 (-13.65, -10.4) -> (-13.0642, -10.4)
  line L35 (-13.0642, -10.4) -> (-10.15, -13.3142)
  line L36 (-15.65, -13.4) -> (-15.65, -18.9)
  line L37 (-15.65, -18.9) -> (-15.9, -18.9)
  line L38 (-15.9, -18.9) -> (-15.9, -13.4)
  line L39 (-15.9, -13.4) -> (-15.65, -13.4)
  line L40 (-15.9, -13.15) -> (-15.9, -19.15) projected
  point P0 (-5.9, 6)
  point P1 (-15.9, -13.4)
  point P2 (-15.9, -18.9)
  dimension "d69" = 0.25
  dimension "d98" = 0.25
  constraints: 44 end point, 16 point on circle, 8 centre point, 3 equal length, 1 collinear, 1 perpendicular, 24 other
  measures "d69" distance between parallel lines of L16 L18
  measures "d98" distance between parallel lines of L6 L26
extrude "Extrusion15" cut sketch "Sketch14" against normal up to surface (2 mm away) contours L9 L8 L7 L6 L5 L4 L3 L2 L1 L37 L30 L29 L28 L27 L26 L35 L34 L33 L32 L39 L0 | L17 A7 L16 A6 L15 A5 L14 A4 L13 A3 L12 A2 L11 A1 L10 A0
fillet "Fillet8" radius 0.5 10 edges at (-10, 18.8, 19.4) (-7.75, 18.8, 19.4) (-7.75, 18.8, 16.4) (-4.25, 18.8, 24.9858) (-7.1642, 18.8, 27.9) (-7.1642, 18.8, 16.4) (-4.25, 18.8, 19.3142) (-7.75, 18.8, 27.9) (-10, 18.8, 24.9) (-7.75, 18.8, 24.9)
fillet "Fillet9" radius 0.5 2 edges at (5.9, 4.4858, 3) (-4.4858, -5.9, 3)
sketch "Sketch15" plane through (0, -5.9, 12.15) normal (0, 0, -1) x (-1, 0, 0)
  line L0 (-9, 23.7) -> (9, 23.7) projected
  line L1 (-9, 18.9) -> (-9, 23.7) projected
  line L2 (-5.9, 18.9) -> (-9, 18.9) projected
  line L3 (-5.9, 18.9) -> (-5.9, 5.9) projected
  arc A0 (-5.9, 5.9) -> (0, 0) centre (0, 5.9) ccw projected
  line L4 (0, 0) -> (13, 0) projected
  line L5 (13, -3.1) -> (13, 0) projected
  line L6 (24.15, -3.1) -> (13, -3.1) projected
  line L7 (24.15, 14.9) -> (24.15, -3.1) projected
  line L8 (13, 14.9) -> (24.15, 14.9) projected
  arc A1 (9, 18.9) -> (13, 14.9) centre (13, 18.9) ccw projected
  line L9 (9, 23.7) -> (9, 18.9) projected
  circle A2 centre (0, 5.9) radius 5.25
  dimension "d74" = 10.5
  constraints: 1 centre point, 1 coincident
  measures "d74" diameter of A2
extrude "Extrusion16" cut sketch "Sketch15" against normal blind 6 contours A2
fillet "Fillet10" radius 0.5 2 edges at (5.25, 0, 12.15) (5.25, 0, 18.15)
sketch "Sketch16" plane through (0, -5.9, 12.15) normal (0, 0, -1) x (-1, 0, 0)
  line L0 (9, 23.7) -> (9, 18.9) projected
  line L1 (-9, 23.7) -> (9, 23.7) projected
  line L2 (-9, 18.9) -> (-9, 23.7) projected
  line L3 (-5.9, 18.9) -> (-9, 18.9) projected
  line L4 (-5.9, 18.9) -> (-5.9, 5.9) projected
  arc A0 (-5.9, 5.9) -> (0, 0) centre (0, 5.9) ccw projected
  line L5 (0, 0) -> (13, 0) projected
  line L6 (13, -3.1) -> (13, 0) projected
  line L7 (24.15, -3.1) -> (13, -3.1) projected
  line L8 (24.15, 14.9) -> (24.15, -3.1) projected
  line L9 (13, 14.9) -> (24.15, 14.9) projected
  arc A1 (9, 18.9) -> (13, 14.9) centre (13, 18.9) ccw projected
  circle A2 centre (0, 5.9) radius 5.75 projected
  line L10 (22.7631, 5.9) -> (20.3816, 1.775)
  line L11 (20.3816, 1.775) -> (15.6184, 1.775)
  line L12 (15.6184, 1.775) -> (13.2369, 5.9)
  line L13 (13.2369, 5.9) -> (15.6184, 10.025)
  line L14 (15.6184, 10.025) -> (20.3816, 10.025)
  line L15 (20.3816, 10.025) -> (22.7631, 5.9)
  line L16 (20.3816, 10.025) -> (24.15, 10.025)
  line L17 (24.15, 10.025) -> (24.15, 1.775)
  line L18 (24.15, 1.775) -> (20.3816, 1.775)
  line L19 (20.3816, 1.775) -> (20.3816, 10.025)
  line L20 (0, 12.6369) -> (-4.125, 15.0184)
  line L21 (-4.125, 15.0184) -> (-4.125, 19.7816)
  line L22 (-4.125, 19.7816) -> (0, 22.1631)
  line L23 (0, 22.1631) -> (4.125, 19.7816)
  line L24 (4.125, 19.7816) -> (4.125, 15.0184)
  line L25 (4.125, 15.0184) -> (0, 12.6369)
  line L26 (4.125, 19.7816) -> (-4.125, 19.7816)
  line L27 (-4.125, 19.7816) -> (-4.125, 23.7)
  line L28 (-4.125, 23.7) -> (4.125, 23.7)
  line L29 (4.125, 23.7) -> (4.125, 19.7816)
  point P0 (18, 5.9)
  point P1 (0, 17.4)
  point P2 (4.125, 23.7)
  point P3 (-4.125, 23.7)
  point P4 (24.15, 1.775)
  point P5 (24.15, 10.025)
  dimension "d78" = 8.25
  dimension "d79" = 18
  dimension "d80" = 11.5
  constraints: 40 end point, 4 parallel, 3 collinear, 3 horizontal, 3 perpendicular, 1 horizontal alignment, 1 vertical, 1 vertical alignment, 26 other
  measures "d78" distance between parallel lines of L14 L11
  measures "d79" distance of point (0, 5.9) point (18, 5.9)
  measures "d80" distance of point (0, 5.9) point (0, 17.4)
ref_plane "Work Plane10" through (0, -5.9, 23.15) normal (0, 0, -1) x (-1, 0, 0)
ref_plane "Work Plane9" through (0, -5.9, 17.15) normal (0, 0, -1) x (-1, 0, 0)
extrude "Extrusion17" cut sketch "Sketch16" against normal up to surface (8 mm away) from surface at -3 contours L19 L11 L12 L13 L14 | L15 L10 L19
extrude "Extrusion18" cut sketch "Sketch16" against normal up to surface (6 mm away) from surface at -5 contours L8 L18 L10 L15 L16
hole "Hole2" at (-18, 0, 12.15) direction (0, 0, 1) diameter 5.2 depth 11
fillet "Fillet11" radius 0.5 6 edges at (-22.2658, -4.125, 17.15) (-22.2658, 4.125, 17.15) (-19.8842, -4.125, 23.15) (-14.4276, -2.0625, 23.15) (-14.4276, 2.0625, 23.15) (-19.8842, 4.125, 23.15)
fillet "Fillet12" radius 0.5 8 edges at (-24.15, 3.9786, 17.2964) (-24.15, 4.125, 20.15) (-24.15, 3.9786, 23.0036) (-24.15, 0, 23.15) (-24.15, -3.9786, 23.0036) (-24.15, -4.125, 20.15) (-24.15, -3.9786, 17.2964) (-24.15, 0, 17.15)
fillet "Fillet13" radius 0.25 35 edges at (-24.15, -7.3839, 27.9) (-24.15, -7.1721, 27.881) (-24.15, -5.7071, 26.4429) (-24.15, -4.269, 24.9779) (-24.15, -4.25, 24.1564) (-24.0752, -4.25, 23.0406) (-23.9807, -4.25, 19.4178) (-23.9807, -4.25, 21.0339) (-24.0021, -4.27, 19.3198) (-24.124, -4.4658, 19.0984) (-24.15, -5.858, 17.7062) (-24.15, -7.1721, 16.419) (-24.15, -7.3839, 16.4) (-24.15, -7.6768, 16.4732) (-24.15, -7.75, 22.15) (-24.15, -7.6768, 27.8268) (-24.15, 5.6465, 26.3823) (-24.15, 7.4414, 27.7408) (-24.15, 7.75, 26.3395) (-24.15, 7.8964, 25.0464) (-24.15, 8.875, 24.9) (-24.15, 9.8536, 24.7536) (-24.15, 4.25, 24.1047) (-24.0752, 4.25, 23.0406) (-23.9807, 4.25, 21.0857) (-24.0227, 4.2917, 19.3213) (-24.136, 4.5074, 19.0568) (-24.15, 5.7608, 17.8034) (-24.15, 7.4414, 16.5592) (-24.15, 7.75, 17.9605) (-24.15, 7.8964, 19.2536) (-24.15, 8.875, 19.4) (-24.15, 9.8536, 19.5464) (-24.15, 4.2881, 24.97) (-24.15, -2.9697, 26.1803)
fillet "Fillet14" radius 0.25 31 edges at (-8.875, 17.8, 24.9) (-9.8536, 17.8, 24.7536) (-7.75, 17.8, 26.3395) (-7.4414, 17.8, 27.7408) (-5.6465, 17.8, 26.3823) (-4.2881, 17.8, 24.97) (-4.25, 17.8, 22.15) (-4.2881, 17.8, 19.33) (-5.6465, 17.8, 17.9177) (-7.4414, 17.8, 16.5592) (-7.75, 17.8, 17.9605) (-7.8964, 17.8, 19.2536) (-8.875, 17.8, 19.4) (-9.8536, 17.8, 19.5464) (-7.8964, 17.8, 25.0464) (-5.6768, 17.8, 29.8268) (0.75, 17.8, 29.9) (7.5303, 17.8, 29.6803) (7.75, 17.8, 22.9) (7.6768, 17.8, 16.4732) (7.3839, 17.8, 16.4) (7.1721, 17.8, 16.419) (5.7071, 17.8, 17.8571) (4.269, 17.8, 19.3221) (4.25, 17.8, 21.2839) (3.2981, 17.8, 25.4481) (-0.8661, 17.8, 26.4) (-2.8279, 17.8, 26.419) (-4.2929, 17.8, 27.8571) (-5.731, 17.8, 29.3221) (-5.75, 17.8, 29.5339)
ref_plane "Work Plane8" through (0, -5.9, 15.15) normal (0, 0, -1) x (-1, 0, 0)
equation "\"d24\" = d21"
equation "\"d42\" = d41"
body "Solid1"
body "Solid2"
